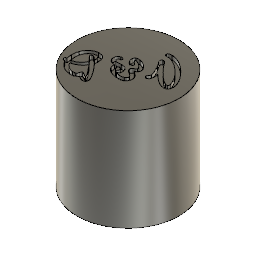
A_and_D_stamp_thick_lines (Autodesk Fusion 360 design; units mm, degrees)
Autodesk Fusion 360 part; units mm, degrees
sketch "Sketch1" plane through (0, 0, 0) normal (0, 0, 1) x (1, 0, 0)
  circle A0 centre (0, 0) radius 12.5
  dimension "d1" = 25
  constraint coincident A0.centre origin
  measures "d1" diameter of A0
extrude "Extrude1" add sketch "Sketch1" along normal blind 25
sketch "Sketch2" plane through (0, 0, 25) normal (0, 0, 1) x (-1, 0, 0)
  circle A0 centre (0, 0) radius 12.5
  spline S0 degree 3 poles (-1.2026, -0.3029) (-1.571, -0.0575) (-1.9494, 0.1661) (-2.255, 0.4915) knots 0 0 0 0 1 1 1 1
  spline S1 degree 3 poles (-2.255, 0.4915) (-2.9403, 1.2218) (-2.7888, 2.5407) (-1.8641, 3.0044) knots 0 0 0 0 1 1 1 1
  spline S2 degree 3 poles (-1.8641, 3.0044) (-1.5783, 3.1479) (-1.1887, 3.1989) (-0.8719, 3.2028) knots 0 0 0 0 1 1 1 1
  spline S3 degree 3 poles (-0.8719, 3.2028) (0.3128, 3.2167) (1.9803, 2.8311) (2.4949, 1.6153) knots 0 0 0 0 1 1 1 1
  spline S4 degree 3 poles (2.4949, 1.6153) (2.6418, 1.2674) (2.6339, 1.0538) (2.6339, 0.6893) knots 0 0 0 0 1 1 1 1
  spline S5 degree 3 poles (2.6339, 0.6893) (3.3317, 0.6827) (3.9515, 0.516) (4.1691, -0.2368) knots 0 0 0 0 1 1 1 1
  spline S6 degree 3 poles (4.1691, -0.2368) (4.3398, -0.8268) (4.1215, -1.5087) (3.4938, -1.7211) knots 0 0 0 0 1 1 1 1
  spline S7 degree 3 poles (3.4938, -1.7211) (3.3648, -1.7455) (3.1637, -1.77) (3.0321, -1.7211) knots 0 0 0 0 1 1 1 1
  spline S8 degree 3 poles (3.0321, -1.7211) (2.696, -1.6536) (2.6451, -1.2944) (2.8058, -1.1641) knots 0 0 0 0 1 1 1 1
  spline S9 degree 3 poles (2.8058, -1.1641) (2.8753, -1.1079) (3.7306, -1.0444) (3.4382, -0.5027) knots 0 0 0 0 1 1 1 1
  spline S10 degree 3 poles (3.4382, -0.5027) (3.4031, -0.4372) (3.3429, -0.371) (3.288, -0.3214) knots 0 0 0 0 1 1 1 1
  spline S11 degree 3 poles (3.288, -0.3214) (2.8852, 0.0437) (2.3203, -0.1647) (1.8401, -0.1706) knots 0 0 0 0 1 1 1 1
  spline S12 degree 3 poles (1.8401, -0.1706) (1.2706, -0.1766) (0.8757, -0.1455) (0.4583, 0.2951) knots 0 0 0 0 1 1 1 1
  spline S13 degree 3 poles (0.4583, 0.2951) (0.0065, 0.7713) (-0.1119, 1.9434) (0.7156, 2.0784) knots 0 0 0 0 1 1 1 1
  spline S14 degree 3 poles (0.7156, 2.0784) (0.0694, 2.4091) (-0.5874, 2.5275) (-1.2687, 2.2173) knots 0 0 0 0 1 1 1 1
  spline S15 degree 3 poles (-1.2687, 2.2173) (-1.5677, 2.081) (-1.9514, 1.7946) (-1.7834, 1.4169) knots 0 0 0 0 1 1 1 1
  spline S16 degree 3 poles (-1.7834, 1.4169) (-1.4804, 0.7363) (-0.0437, 0.4955) (-0.1542, -0.3029) knots 0 0 0 0 1 1 1 1
  spline S17 degree 3 poles (-0.1542, -0.3029) (-0.2316, -0.8651) (-0.9942, -0.8122) (-1.0822, -1.2316) knots 0 0 0 0 1 1 1 1
  spline S18 degree 3 poles (-1.0822, -1.2316) (-1.1292, -1.4538) (-0.8725, -1.7402) (-0.7336, -1.8904) knots 0 0 0 0 1 1 1 1
  spline S19 degree 3 poles (-0.7336, -1.8904) (-0.2693, -2.3898) (0.3386, -2.8178) (1.0464, -2.7503) knots 0 0 0 0 1 1 1 1
  spline S20 degree 3 poles (1.0464, -2.7503) (0.7851, -2.0842) (0.2678, -2.0392) (0.164, -1.6893) knots 0 0 0 0 1 1 1 1
  spline S21 degree 3 poles (0.164, -1.6893) (0.0753, -1.3917) (0.4008, -1.1463) (0.7156, -1.1754) knots 0 0 0 0 1 1 1 1
  spline S22 degree 3 poles (0.7156, -1.1754) (0.9683, -1.1985) (1.1178, -1.3745) (1.2666, -1.5597) knots 0 0 0 0 1 1 1 1
  spline S23 degree 3 poles (1.2666, -1.5597) (1.3916, -1.7158) (1.5716, -1.9698) (1.6423, -2.155) knots 0 0 0 0 1 1 1 1
  spline S24 degree 3 poles (1.6423, -2.155) (1.7826, -2.5234) (1.7627, -3.1088) (1.3744, -3.3158) knots 0 0 0 0 1 1 1 1
  spline S25 degree 3 poles (1.3744, -3.3158) (1.1528, -3.4336) (0.7004, -3.427) (0.451, -3.4005) knots 0 0 0 0 1 1 1 1
  spline S26 degree 3 poles (0.451, -3.4005) (-0.3771, -3.3112) (-1.2787, -2.7252) (-1.7139, -2.0227) knots 0 0 0 0 1 1 1 1
  spline S27 degree 3 poles (-1.7139, -2.0227) (-2.1809, -1.2686) (-2.0883, -0.6211) (-1.2026, -0.3029) knots 0 0 0 0 1 1 1 1
  spline S28 degree 3 poles (1.1125, 1.8799) (1.0702, 1.3587) (0.8228, 1.3474) (0.8307, 1.0888) knots 0 0 0 0 1 1 1 1
  spline S29 degree 3 poles (0.8307, 1.0888) (0.8426, 0.7184) (1.8229, 0.3936) (1.809, 0.9552) knots 0 0 0 0 1 1 1 1
  spline S30 degree 3 poles (1.809, 0.9552) (1.807, 1.0379) (1.7713, 1.143) (1.7389, 1.2185) knots 0 0 0 0 1 1 1 1
  spline S31 degree 3 poles (1.7389, 1.2185) (1.6919, 1.3289) (1.6159, 1.4533) (1.5405, 1.5465) knots 0 0 0 0 1 1 1 1
  spline S32 degree 3 poles (1.5405, 1.5465) (1.3976, 1.7225) (1.3056, 1.7754) (1.1125, 1.8799) knots 0 0 0 0 1 1 1 1
  line L0 (1.1125, 1.8799) -> (1.1125, 1.9461)
  line L1 (1.1125, 1.9461) -> (1.0464, 1.8799)
  line L2 (1.0464, 1.8799) -> (1.1125, 1.8799)
extrude "Extrude2" cut sketch "Sketch2" against normal blind 1 contours S0 S1 S2 S3 S4 S5 S6 S7 S8 S9 S10 S11 S12 S13 S14 S15 S16 S17 S18 S19 S20 S21 S22 S23 S24 S25 S26 S27
sketch "Sketch3" plane through (0, 0, 25) normal (0, 0, 1) x (-1, 0, 0)
  circle A0 centre (0, 0) radius 12.5
  spline S0 degree 3 poles (1.3744, -3.3158) (1.1528, -3.4336) (0.7004, -3.427) (0.451, -3.4005) knots 0 0 0 0 1 1 1 1
  spline S1 degree 3 poles (0.451, -3.4005) (-0.3771, -3.3112) (-1.2787, -2.7252) (-1.7139, -2.0227) knots 0 0 0 0 1 1 1 1
  spline S2 degree 3 poles (-1.7139, -2.0227) (-2.1809, -1.2686) (-2.0883, -0.6211) (-1.2026, -0.3029) knots 0 0 0 0 1 1 1 1
  spline S3 degree 3 poles (-1.2026, -0.3029) (-1.571, -0.0575) (-1.9494, 0.1661) (-2.255, 0.4915) knots 0 0 0 0 1 1 1 1
  spline S4 degree 3 poles (-2.255, 0.4915) (-2.9403, 1.2218) (-2.7888, 2.5407) (-1.8641, 3.0044) knots 0 0 0 0 1 1 1 1
  spline S5 degree 3 poles (-1.8641, 3.0044) (-1.5783, 3.1479) (-1.1887, 3.1989) (-0.8719, 3.2028) knots 0 0 0 0 1 1 1 1
  spline S6 degree 3 poles (-0.8719, 3.2028) (0.3128, 3.2167) (1.9803, 2.8311) (2.4949, 1.6153) knots 0 0 0 0 1 1 1 1
  spline S7 degree 3 poles (2.4949, 1.6153) (2.6418, 1.2674) (2.6339, 1.0538) (2.6339, 0.6893) knots 0 0 0 0 1 1 1 1
  spline S8 degree 3 poles (2.6339, 0.6893) (3.3317, 0.6827) (3.9515, 0.516) (4.1691, -0.2368) knots 0 0 0 0 1 1 1 1
  spline S9 degree 3 poles (4.1691, -0.2368) (4.3398, -0.8268) (4.1215, -1.5087) (3.4938, -1.7211) knots 0 0 0 0 1 1 1 1
  spline S10 degree 3 poles (3.4938, -1.7211) (3.3648, -1.7455) (3.1637, -1.77) (3.0321, -1.7211) knots 0 0 0 0 1 1 1 1
  spline S11 degree 3 poles (3.0321, -1.7211) (2.696, -1.6536) (2.6451, -1.2944) (2.8058, -1.1641) knots 0 0 0 0 1 1 1 1
  spline S12 degree 3 poles (2.8058, -1.1641) (2.8753, -1.1079) (3.7306, -1.0444) (3.4382, -0.5027) knots 0 0 0 0 1 1 1 1
  spline S13 degree 3 poles (3.4382, -0.5027) (3.4031, -0.4372) (3.3429, -0.371) (3.288, -0.3214) knots 0 0 0 0 1 1 1 1
  spline S14 degree 3 poles (3.288, -0.3214) (2.8852, 0.0437) (2.3203, -0.1647) (1.8401, -0.1706) knots 0 0 0 0 1 1 1 1
  spline S15 degree 3 poles (1.8401, -0.1706) (1.2706, -0.1766) (0.8757, -0.1455) (0.4583, 0.2951) knots 0 0 0 0 1 1 1 1
  spline S16 degree 3 poles (0.4583, 0.2951) (0.0065, 0.7713) (-0.1119, 1.9434) (0.7156, 2.0784) knots 0 0 0 0 1 1 1 1
  spline S17 degree 3 poles (0.7156, 2.0784) (0.0694, 2.4091) (-0.5874, 2.5275) (-1.2687, 2.2173) knots 0 0 0 0 1 1 1 1
  spline S18 degree 3 poles (-1.2687, 2.2173) (-1.5677, 2.081) (-1.9514, 1.7946) (-1.7834, 1.4169) knots 0 0 0 0 1 1 1 1
  spline S19 degree 3 poles (-1.7834, 1.4169) (-1.4804, 0.7363) (-0.0437, 0.4955) (-0.1542, -0.3029) knots 0 0 0 0 1 1 1 1
  spline S20 degree 3 poles (-0.1542, -0.3029) (-0.2316, -0.8651) (-0.9942, -0.8122) (-1.0822, -1.2316) knots 0 0 0 0 1 1 1 1
  spline S21 degree 3 poles (-1.0822, -1.2316) (-1.1292, -1.4538) (-0.8725, -1.7402) (-0.7336, -1.8904) knots 0 0 0 0 1 1 1 1
  spline S22 degree 3 poles (-0.7336, -1.8904) (-0.2693, -2.3898) (0.3386, -2.8178) (1.0464, -2.7503) knots 0 0 0 0 1 1 1 1
  spline S23 degree 3 poles (1.0464, -2.7503) (0.7851, -2.0842) (0.2678, -2.0392) (0.164, -1.6893) knots 0 0 0 0 1 1 1 1
  spline S24 degree 3 poles (0.164, -1.6893) (0.0753, -1.3917) (0.4008, -1.1463) (0.7156, -1.1754) knots 0 0 0 0 1 1 1 1
  spline S25 degree 3 poles (0.7156, -1.1754) (0.9683, -1.1985) (1.1178, -1.3745) (1.2666, -1.5597) knots 0 0 0 0 1 1 1 1
  spline S26 degree 3 poles (1.2666, -1.5597) (1.3916, -1.7158) (1.5716, -1.9698) (1.6423, -2.155) knots 0 0 0 0 1 1 1 1
  spline S27 degree 3 poles (1.6423, -2.155) (1.7826, -2.5234) (1.7627, -3.1088) (1.3744, -3.3158) knots 0 0 0 0 1 1 1 1
  spline S28 degree 3 poles (-4.8406, -2.4634) (-4.9248, -1.8268) (-5.0859, -0.5314) (-4.2056, -0.3465) knots 0 0 0 0 1 1 1 1
  spline S29 degree 3 poles (-4.2056, -0.3465) (-3.9389, -0.2909) (-3.6738, -0.4187) (-3.673, -0.7172) knots 0 0 0 0 1 1 1 1
  spline S30 degree 3 poles (-3.673, -0.7172) (-3.6722, -1.1029) (-4.0881, -1.1609) (-4.0762, -1.6697) knots 0 0 0 0 1 1 1 1
  spline S31 degree 3 poles (-4.0762, -1.6697) (-4.0627, -2.2682) (-3.3412, -3.689) (-3.0079, -4.2097) knots 0 0 0 0 1 1 1 1
  line L0 (-3.0079, -4.2097) -> (-2.253, -5.3209)
  spline S32 degree 3 poles (-2.253, -5.3209) (-2.0831, -5.6019) (-1.903, -6.1099) (-2.3848, -6.1822) knots 0 0 0 0 1 1 1 1
  spline S33 degree 3 poles (-2.3848, -6.1822) (-3.0166, -6.2766) (-3.3373, -5.5146) (-3.6683, -5.0828) knots 0 0 0 0 1 1 1 1
  spline S34 degree 3 poles (-3.6683, -5.0828) (-4.3398, -4.2097) (-5.7868, -2.777) (-6.6662, -2.1007) knots 0 0 0 0 1 1 1 1
  spline S35 degree 3 poles (-6.6662, -2.1007) (-6.929, -1.8983) (-7.4814, -1.5292) (-7.7775, -1.3982) knots 0 0 0 0 1 1 1 1
  spline S36 degree 3 poles (-7.7775, -1.3982) (-7.9593, -1.3165) (-8.1895, -1.2355) (-8.3538, -1.3982) knots 0 0 0 0 1 1 1 1
  spline S37 degree 3 poles (-8.3538, -1.3982) (-8.5268, -1.5736) (-8.4673, -1.8578) (-8.4109, -2.0666) knots 0 0 0 0 1 1 1 1
  spline S38 degree 3 poles (-8.4109, -2.0666) (-8.2768, -2.569) (-7.9005, -3.3072) (-7.6021, -3.7334) knots 0 0 0 0 1 1 1 1
  spline S39 degree 3 poles (-7.6021, -3.7334) (-6.6758, -5.0582) (-5.2724, -6.3512) (-3.8087, -7.0569) knots 0 0 0 0 1 1 1 1
  spline S40 degree 3 poles (-3.8087, -7.0569) (-3.4397, -7.2347) (-2.8674, -7.441) (-2.4594, -7.4609) knots 0 0 0 0 1 1 1 1
  spline S41 degree 3 poles (-2.4594, -7.4609) (-2.2411, -7.4712) (-1.7283, -7.4093) (-1.5886, -7.5911) knots 0 0 0 0 1 1 1 1
  spline S42 degree 3 poles (-1.5886, -7.5911) (-1.5172, -7.6831) (-1.5156, -7.8292) (-1.5426, -7.9371) knots 0 0 0 0 1 1 1 1
  spline S43 degree 3 poles (-1.5426, -7.9371) (-1.6505, -8.3689) (-2.1054, -8.3443) (-2.4594, -8.3364) knots 0 0 0 0 1 1 1 1
  spline S44 degree 3 poles (-2.4594, -8.3364) (-4.693, -8.2856) (-6.9599, -6.2099) (-8.2244, -4.5272) knots 0 0 0 0 1 1 1 1
  spline S45 degree 3 poles (-8.2244, -4.5272) (-8.8268, -3.7239) (-9.3769, -2.7778) (-9.4372, -1.7491) knots 0 0 0 0 1 1 1 1
  spline S46 degree 3 poles (-9.4372, -1.7491) (-9.5031, -0.6092) (-8.8173, -0.2179) (-7.7775, -0.4537) knots 0 0 0 0 1 1 1 1
  spline S47 degree 3 poles (-7.7775, -0.4537) (-6.8226, -0.6696) (-5.5455, -1.7911) (-4.8406, -2.4634) knots 0 0 0 0 1 1 1 1
  line L1 (-4.7613, -2.5428) -> (-4.7613, -2.4634)
  line L2 (-4.7613, -2.4634) -> (-4.8406, -2.5428)
  line L3 (-4.8406, -2.5428) -> (-4.7613, -2.5428)
extrude "Extrude3" cut sketch "Sketch3" against normal blind 1 contours S28 S29 S30 S31 L0 S32 S33 S34 S35 S36 S37 S38 S39 S40 S41 S42 S43 S44 S45 S46 S47
sketch "Sketch4" plane through (0, 0, 25) normal (0, 0, 1) x (-1, 0, 0)
  spline S0 degree 3 poles (1.3744, -3.3158) (1.1528, -3.4336) (0.7004, -3.427) (0.451, -3.4005) knots 0 0 0 0 1 1 1 1
  spline S1 degree 3 poles (0.451, -3.4005) (-0.3771, -3.3112) (-1.2787, -2.7252) (-1.7139, -2.0227) knots 0 0 0 0 1 1 1 1
  spline S2 degree 3 poles (-1.7139, -2.0227) (-2.1809, -1.2686) (-2.0883, -0.6211) (-1.2026, -0.3029) knots 0 0 0 0 1 1 1 1
  spline S3 degree 3 poles (-1.2026, -0.3029) (-1.571, -0.0575) (-1.9494, 0.1661) (-2.255, 0.4915) knots 0 0 0 0 1 1 1 1
  spline S4 degree 3 poles (-2.255, 0.4915) (-2.9403, 1.2218) (-2.7888, 2.5407) (-1.8641, 3.0044) knots 0 0 0 0 1 1 1 1
  spline S5 degree 3 poles (-1.8641, 3.0044) (-1.5783, 3.1479) (-1.1887, 3.1989) (-0.8719, 3.2028) knots 0 0 0 0 1 1 1 1
  spline S6 degree 3 poles (-0.8719, 3.2028) (0.3128, 3.2167) (1.9803, 2.8311) (2.4949, 1.6153) knots 0 0 0 0 1 1 1 1
  spline S7 degree 3 poles (2.4949, 1.6153) (2.6418, 1.2674) (2.6339, 1.0538) (2.6339, 0.6893) knots 0 0 0 0 1 1 1 1
  spline S8 degree 3 poles (2.6339, 0.6893) (3.3317, 0.6827) (3.9515, 0.516) (4.1691, -0.2368) knots 0 0 0 0 1 1 1 1
  spline S9 degree 3 poles (4.1691, -0.2368) (4.3398, -0.8268) (4.1215, -1.5087) (3.4938, -1.7211) knots 0 0 0 0 1 1 1 1
  spline S10 degree 3 poles (3.4938, -1.7211) (3.3648, -1.7455) (3.1637, -1.77) (3.0321, -1.7211) knots 0 0 0 0 1 1 1 1
  spline S11 degree 3 poles (3.0321, -1.7211) (2.696, -1.6536) (2.6451, -1.2944) (2.8058, -1.1641) knots 0 0 0 0 1 1 1 1
  spline S12 degree 3 poles (2.8058, -1.1641) (2.8753, -1.1079) (3.7306, -1.0444) (3.4382, -0.5027) knots 0 0 0 0 1 1 1 1
  spline S13 degree 3 poles (3.4382, -0.5027) (3.4031, -0.4372) (3.3429, -0.371) (3.288, -0.3214) knots 0 0 0 0 1 1 1 1
  spline S14 degree 3 poles (3.288, -0.3214) (2.8852, 0.0437) (2.3203, -0.1647) (1.8401, -0.1706) knots 0 0 0 0 1 1 1 1
  spline S15 degree 3 poles (1.8401, -0.1706) (1.2706, -0.1766) (0.8757, -0.1455) (0.4583, 0.2951) knots 0 0 0 0 1 1 1 1
  spline S16 degree 3 poles (0.4583, 0.2951) (0.0065, 0.7713) (-0.1119, 1.9434) (0.7156, 2.0784) knots 0 0 0 0 1 1 1 1
  spline S17 degree 3 poles (0.7156, 2.0784) (0.0694, 2.4091) (-0.5874, 2.5275) (-1.2687, 2.2173) knots 0 0 0 0 1 1 1 1
  spline S18 degree 3 poles (-1.2687, 2.2173) (-1.5677, 2.081) (-1.9514, 1.7946) (-1.7834, 1.4169) knots 0 0 0 0 1 1 1 1
  spline S19 degree 3 poles (-1.7834, 1.4169) (-1.4804, 0.7363) (-0.0437, 0.4955) (-0.1542, -0.3029) knots 0 0 0 0 1 1 1 1
  spline S20 degree 3 poles (-0.1542, -0.3029) (-0.2316, -0.8651) (-0.9942, -0.8122) (-1.0822, -1.2316) knots 0 0 0 0 1 1 1 1
  spline S21 degree 3 poles (-1.0822, -1.2316) (-1.1292, -1.4538) (-0.8725, -1.7402) (-0.7336, -1.8904) knots 0 0 0 0 1 1 1 1
  spline S22 degree 3 poles (-0.7336, -1.8904) (-0.2693, -2.3898) (0.3386, -2.8178) (1.0464, -2.7503) knots 0 0 0 0 1 1 1 1
  spline S23 degree 3 poles (1.0464, -2.7503) (0.7851, -2.0842) (0.2678, -2.0392) (0.164, -1.6893) knots 0 0 0 0 1 1 1 1
  spline S24 degree 3 poles (0.164, -1.6893) (0.0753, -1.3917) (0.4008, -1.1463) (0.7156, -1.1754) knots 0 0 0 0 1 1 1 1
  spline S25 degree 3 poles (0.7156, -1.1754) (0.9683, -1.1985) (1.1178, -1.3745) (1.2666, -1.5597) knots 0 0 0 0 1 1 1 1
  spline S26 degree 3 poles (1.2666, -1.5597) (1.3916, -1.7158) (1.5716, -1.9698) (1.6423, -2.155) knots 0 0 0 0 1 1 1 1
  spline S27 degree 3 poles (1.6423, -2.155) (1.7826, -2.5234) (1.7627, -3.1088) (1.3744, -3.3158) knots 0 0 0 0 1 1 1 1
  circle A0 centre (0, 0) radius 12.5
  spline S28 degree 3 poles (-8.2244, -4.5272) (-8.8268, -3.7239) (-9.3769, -2.7778) (-9.4372, -1.7491) knots 0 0 0 0 1 1 1 1
  spline S29 degree 3 poles (-9.4372, -1.7491) (-9.5031, -0.6092) (-8.8173, -0.2179) (-7.7775, -0.4537) knots 0 0 0 0 1 1 1 1
  spline S30 degree 3 poles (-7.7775, -0.4537) (-6.8226, -0.6696) (-5.5455, -1.7911) (-4.8406, -2.4634) knots 0 0 0 0 1 1 1 1
  spline S31 degree 3 poles (-4.8406, -2.4634) (-4.9248, -1.8268) (-5.0859, -0.5314) (-4.2056, -0.3465) knots 0 0 0 0 1 1 1 1
  spline S32 degree 3 poles (-4.2056, -0.3465) (-3.9389, -0.2909) (-3.6738, -0.4187) (-3.673, -0.7172) knots 0 0 0 0 1 1 1 1
  spline S33 degree 3 poles (-3.673, -0.7172) (-3.6722, -1.1029) (-4.0881, -1.1609) (-4.0762, -1.6697) knots 0 0 0 0 1 1 1 1
  spline S34 degree 3 poles (-4.0762, -1.6697) (-4.0627, -2.2682) (-3.3412, -3.689) (-3.0079, -4.2097) knots 0 0 0 0 1 1 1 1
  line L0 (-3.0079, -4.2097) -> (-2.253, -5.3209)
  spline S35 degree 3 poles (-2.253, -5.3209) (-2.0831, -5.6019) (-1.903, -6.1099) (-2.3848, -6.1822) knots 0 0 0 0 1 1 1 1
  spline S36 degree 3 poles (-2.3848, -6.1822) (-3.0166, -6.2766) (-3.3373, -5.5146) (-3.6683, -5.0828) knots 0 0 0 0 1 1 1 1
  spline S37 degree 3 poles (-3.6683, -5.0828) (-4.3398, -4.2097) (-5.7868, -2.777) (-6.6662, -2.1007) knots 0 0 0 0 1 1 1 1
  spline S38 degree 3 poles (-6.6662, -2.1007) (-6.929, -1.8983) (-7.4814, -1.5292) (-7.7775, -1.3982) knots 0 0 0 0 1 1 1 1
  spline S39 degree 3 poles (-7.7775, -1.3982) (-7.9593, -1.3165) (-8.1895, -1.2355) (-8.3538, -1.3982) knots 0 0 0 0 1 1 1 1
  spline S40 degree 3 poles (-8.3538, -1.3982) (-8.5268, -1.5736) (-8.4673, -1.8578) (-8.4109, -2.0666) knots 0 0 0 0 1 1 1 1
  spline S41 degree 3 poles (-8.4109, -2.0666) (-8.2768, -2.569) (-7.9005, -3.3072) (-7.6021, -3.7334) knots 0 0 0 0 1 1 1 1
  spline S42 degree 3 poles (-7.6021, -3.7334) (-6.6758, -5.0582) (-5.2724, -6.3512) (-3.8087, -7.0569) knots 0 0 0 0 1 1 1 1
  spline S43 degree 3 poles (-3.8087, -7.0569) (-3.4397, -7.2347) (-2.8674, -7.441) (-2.4594, -7.4609) knots 0 0 0 0 1 1 1 1
  spline S44 degree 3 poles (-2.4594, -7.4609) (-2.2411, -7.4712) (-1.7283, -7.4093) (-1.5886, -7.5911) knots 0 0 0 0 1 1 1 1
  spline S45 degree 3 poles (-1.5886, -7.5911) (-1.5172, -7.6831) (-1.5156, -7.8292) (-1.5426, -7.9371) knots 0 0 0 0 1 1 1 1
  spline S46 degree 3 poles (-1.5426, -7.9371) (-1.6505, -8.3689) (-2.1054, -8.3443) (-2.4594, -8.3364) knots 0 0 0 0 1 1 1 1
  spline S47 degree 3 poles (-2.4594, -8.3364) (-4.693, -8.2856) (-6.9599, -6.2099) (-8.2244, -4.5272) knots 0 0 0 0 1 1 1 1
  line L1 (9.8362, 5.1157) -> (9.995, 3.8457)
  spline S48 degree 3 poles (9.995, 3.8457) (10.0006, 3.3448) (9.9109, 2.7281) (9.7354, 2.2582) knots 0 0 0 0 1 1 1 1
  spline S49 degree 3 poles (9.7354, 2.2582) (9.3473, 1.2184) (8.3067, 0.1309) (7.1375, 0.1151) knots 0 0 0 0 1 1 1 1
  spline S50 degree 3 poles (7.1375, 0.1151) (6.4017, 0.1055) (5.9889, 0.0833) (5.5111, 0.7501) knots 0 0 0 0 1 1 1 1
  spline S51 degree 3 poles (5.5111, 0.7501) (5.1888, 1.1993) (5.2134, 1.8089) (5.2293, 2.3376) knots 0 0 0 0 1 1 1 1
  spline S52 degree 3 poles (5.2293, 2.3376) (5.2444, 2.5416) (5.3055, 2.7836) (5.2293, 2.9726) knots 0 0 0 0 1 1 1 1
  spline S53 degree 3 poles (5.2293, 2.9726) (5.1555, 3.1321) (4.5935, 3.7449) (4.4388, 3.9251) knots 0 0 0 0 1 1 1 1
  spline S54 degree 3 poles (4.4388, 3.9251) (3.8831, 4.572) (3.3688, 5.2514) (2.9417, 5.9888) knots 0 0 0 0 1 1 1 1
  spline S55 degree 3 poles (2.9417, 5.9888) (2.729, 6.3563) (2.4917, 6.7476) (2.4623, 7.1794) knots 0 0 0 0 1 1 1 1
  spline S56 degree 3 poles (2.4623, 7.1794) (2.4242, 7.7232) (2.5203, 7.97) (3.0894, 7.9724) knots 0 0 0 0 1 1 1 1
  spline S57 degree 3 poles (3.0894, 7.9724) (3.2894, 7.9732) (3.4553, 7.966) (3.645, 7.8946) knots 0 0 0 0 1 1 1 1
  spline S58 degree 3 poles (3.645, 7.8946) (3.9212, 7.7898) (4.1752, 7.5588) (4.3372, 7.5493) knots 0 0 0 0 1 1 1 1
  spline S59 degree 3 poles (4.3372, 7.5493) (4.5888, 7.5334) (4.7547, 7.9105) (5.2325, 8.0708) knots 0 0 0 0 1 1 1 1
  spline S60 degree 3 poles (5.2325, 8.0708) (5.4008, 8.128) (5.5349, 8.1288) (5.7088, 8.1319) knots 0 0 0 0 1 1 1 1
  spline S61 degree 3 poles (5.7088, 8.1319) (6.5684, 8.1454) (6.8946, 8.1375) (7.6931, 7.7454) knots 0 0 0 0 1 1 1 1
  spline S62 degree 3 poles (7.6931, 7.7454) (8.1979, 7.4977) (8.6583, 7.1366) (9.0163, 6.7032) knots 0 0 0 0 1 1 1 1
  line L2 (9.0163, 6.7032) -> (9.4894, 6.0364)
  spline S63 degree 3 poles (9.4894, 6.0364) (9.7347, 5.8221) (10.1117, 5.9983) (10.2069, 5.588) knots 0 0 0 0 1 1 1 1
  spline S64 degree 3 poles (10.2069, 5.588) (10.2831, 5.2562) (10.1133, 5.1641) (9.8362, 5.1157) knots 0 0 0 0 1 1 1 1
  spline S65 degree 3 poles (8.8837, 5.1157) (7.5169, 4.8712) (7.12, 4.2156) (6.3437, 3.2107) knots 0 0 0 0 1 1 1 1
  line L3 (6.3437, 3.2107) -> (7.528, 1.9335)
  spline S66 degree 3 poles (7.528, 1.9335) (7.6685, 1.6208) (7.3597, 1.3652) (7.0581, 1.4144) knots 0 0 0 0 1 1 1 1
  spline S67 degree 3 poles (7.0581, 1.4144) (6.7732, 1.4613) (6.3096, 1.9756) (6.0262, 2.1788) knots 0 0 0 0 1 1 1 1
  spline S68 degree 3 poles (6.0262, 2.1788) (6.027, 1.9272) (6.0143, 1.7065) (6.1032, 1.4644) knots 0 0 0 0 1 1 1 1
  spline S69 degree 3 poles (6.1032, 1.4644) (6.5057, 0.3691) (7.8027, 1.1247) (8.3115, 1.7034) knots 0 0 0 0 1 1 1 1
  spline S70 degree 3 poles (8.3115, 1.7034) (9.1663, 2.6765) (9.1997, 3.9251) (8.8837, 5.1157) knots 0 0 0 0 1 1 1 1
  spline S71 degree 3 poles (5.7881, 3.9251) (6.3723, 4.9252) (7.3724, 5.5753) (8.4869, 5.8301) knots 0 0 0 0 1 1 1 1
  spline S72 degree 3 poles (8.4869, 5.8301) (8.0924, 6.5651) (7.1248, 7.3072) (6.2644, 7.3366) knots 0 0 0 0 1 1 1 1
  spline S73 degree 3 poles (6.2644, 7.3366) (6.054, 7.3437) (5.7437, 7.3493) (5.5587, 7.2453) knots 0 0 0 0 1 1 1 1
  spline S74 degree 3 poles (5.5587, 7.2453) (5.0261, 6.9453) (5.4301, 6.2507) (4.9102, 6.1833) knots 0 0 0 0 1 1 1 1
  spline S75 degree 3 poles (4.9102, 6.1833) (4.503, 6.1293) (4.1276, 6.7286) (3.4862, 6.9413) knots 0 0 0 0 1 1 1 1
  spline S76 degree 3 poles (3.4862, 6.9413) (3.768, 6.0499) (5.0595, 4.7315) (5.6294, 3.9251) knots 0 0 0 0 1 1 1 1
  line L4 (5.6294, 3.9251) -> (5.7881, 3.9251)
  line L5 (3.4863, 6.9413) -> (3.4862, 7.0207)
  line L6 (3.4862, 7.0207) -> (3.4069, 6.9413)
  line L7 (3.4069, 6.9413) -> (3.4863, 6.9413)
  line L8 (3.4069, 7.0207) -> (3.4069, 7.1001)
  line L9 (3.4069, 7.1001) -> (3.3275, 7.0207)
  line L10 (3.3275, 7.0207) -> (3.4069, 7.0207)
extrude "Extrude4" cut sketch "Sketch4" against normal blind 1 contours L1 S48 S49 S50 S51 S52 S53 S54 S55 S56 S57 S58 S59 S60 S61 S62 L2 S63 S64
